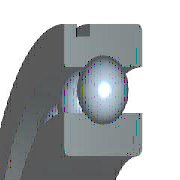
# Autodesk Inventor part: 滚动轴承 6200 N GB/T 276-94
Saved by Autodesk Inventor 2015 (Build 190159000, 159)
## iProperties
Created: 2014-02-16
Part Number: 滚动轴承 6200 N GB/T 276-94
Material: 钢，软
Description: 滚动轴承 - 深沟球轴承 - 外形尺寸
Document SubType Name: Modeling
Standard: GB/T 276-1994
Designer: Administrator
Standard Revision: 1994
Standards Organization: GB
Language: zh-CN
Size Designation: 6200 N
Categories: <MemberInstance><Categories><Category DisplayName="轴用零件" InternalName="7f7aeb1f-a693-4053-b835-cee3144e0d98" Mnemonic="SHFT"><Category DisplayName="轴承" InternalName="242d30a3-7172-44e6-a363-b0a3d8f1b556" Mnemonic="BRNG"><CategoryParameter DisplayName="宽度" InternalName="25fc5f6e-338b-4801-b5ed-8959743e396e" Mnemonic="wdth"/><CategoryParameter DisplayName="尺寸规格" InternalName="2c4e891a-c8f4-49ed-a5c1-5131476c6feb" Mnemonic="sizedes"/><CategoryParameter DisplayName="额定基本动态载荷" InternalName="440972dd-7009-4861-bd45-69ffbb461423" Mnemonic="bdynlrat"/><CategoryParameter DisplayName="轴直径" InternalName="91302473-2833-4451-a660-c5d4a8d6a031" Mnemonic="shaftdia"/><CategoryParameter DisplayName="接触角" InternalName="aa21a452-7974-4a55-b5cf-1c2972de2aea" Mnemonic="TouchAngle"/><CategoryParameter DisplayName="外径" InternalName="d441686c-04bd-4681-b674-94fbc173ec23" Mnemonic="outdia"/><Category DisplayName="球轴承" InternalName="9b553946-0899-4a5e-a403-c1d9295e77c1" Mnemonic="BALLBEAR"><CategoryParameter DisplayName="当 Fa/Fr &lt;= e 时的径向动态载荷系数" InternalName="051e59b3-bd55-4dad-8b07-38b5cb912881" Mnemonic="raddynfc1"/><CategoryParameter DisplayName="基本额定静载荷" InternalName="0f13fbbf-c511-4d43-b4c7-197b47424baf" Mnemonic="bstatlrat"/><CategoryParameter DisplayName="确定寿命的指数" InternalName="3029e2ef-9460-4be8-bdfd-dfe61437473d" Mnemonic="lifeexp"/><CategoryParameter DisplayName="摩擦系数" InternalName="3086b0f2-3d69-46ff-8a75-fe12e395bb47" Mnemonic="fricfct"/><CategoryParameter DisplayName="最小轴径" InternalName="4a5be9bc-ad86-4bf2-8167-102dad5d3e27" Mnemonic="minshaftdia"/><CategoryParameter DisplayName="当 Fa/Fr &gt; e 时的轴向动态载荷系数" InternalName="4b6ff741-5956-4a40-80f5-34eb9259f88c" Mnemonic="axdynfc2"/><CategoryParameter DisplayName="极限速度 (润滑脂)" InternalName="5237843b-2c8d-46d3-8227-f3e9dd85a12e" Mnemonic="lubgrsp"/><CategoryParameter DisplayName="极限速度 (润滑油)" InternalName="60628548-8907-44dc-8e09-603d72f5766f" Mnemonic="oilspd"/><CategoryParameter DisplayName="轴向静态载荷系数" InternalName="74dbf5e2-8362-409a-802f-3c2235668d99" Mnemonic="axdynfc0"/><CategoryParameter DisplayName="质量" InternalName="7b80f85c-da81-4dea-b8db-d7c689da91b2" Mnemonic="mass"/><CategoryParameter DisplayName="半径" InternalName="83352640-dfae-4cba-bc9f-11ecbfb0001c" Mnemonic="rad"/><CategoryParameter DisplayName="径向静态载荷系数" InternalName="83ce084d-c51e-4598-a871-e8e1e34b26ee" Mnemonic="raddynfc0"/><CategoryParameter DisplayName="当 Fa/Fr &lt;= e 时的轴向动态载荷系数" InternalName="ae45a7db-08df-4411-99a8-2f035015bff9" Mnemonic="axdynfc1"/><CategoryParameter DisplayName="最大安装孔肩直径" InternalName="b5cf89e0-ca87-439c-b08c-a25e2999ab06" Mnemonic="maxhubdia"/><CategoryParameter DisplayName="确定系数的极限值" InternalName="be0ce6fc-cad4-4218-b484-c34dd2571812" Mnemonic="limvalfac"/><CategoryParameter DisplayName="当 Fa/Fr &gt; e 时的径向动态载荷系数" InternalName="e513bdb7-139f-4b3c-af32-49e0ba1226b9" Mnemonic="raddynfc2"/><CategoryParameter DisplayName="最大阶梯圆角半径" InternalName="f6ce6695-cf2c-4ec9-8d20-66671e0e35a4" Mnemonic="maxstprad"/><Category DisplayName="深沟球轴承" InternalName="6f040212-0f73-4fa8-b5e4-17d6525fdc38" Mnemonic="BBDGBB"/></Category></Category></Category><Category DisplayName="数据类型" InternalName="23b78d0f-2648-40c6-8793-ca6db495c9e8" Mnemonic="DATATYPE"><CategoryParameter DisplayName="显示名" InternalName="05415f3d-3907-474b-a020-eb9d644f4cf3" Mnemonic="DISPLAYNAME"/><CategoryParameter DisplayName="标准" InternalName="0c0a119c-1e12-4c84-803f-101930972f5e" Mnemonic="STANDARD"/><CategoryParameter DisplayName="描述" InternalName="13903e3d-64b1-4950-80da-f627842ea37f" Mnemonic="DESCRIPTION"/><CategoryParameter DisplayName="规格" InternalName="2675968c-4ce5-49e0-a4f5-552d29089031" Mnemonic="DESIGNATION"/><CategoryParameter DisplayName="默认列" InternalName="2af9ec52-faaa-4026-b378-f9fa4afca842" Mnemonic="DEFAULTROW"/><CategoryParameter DisplayName="文件夹名称" InternalName="3f06958e-8713-4116-9be7-ed6184ecc97b" Mnemonic="FOLDERNAME"/><CategoryParameter DisplayName="版本指南" InternalName="45a75005-10b1-4dfc-8d6d-dfe629f0b93c" Mnemonic="REVISIONGUID"/><CategoryParameter DisplayName="文件名" InternalName="8b46a4cc-9585-4fed-90c3-899f57e09a73" Mnemonic="FILENAME"/><CategoryParameter DisplayName="标准组织" InternalName="8f5914e1-4693-403f-8ab5-d37768198c9d" Mnemonic="STDSORG"/><CategoryParameter DisplayName="系列版本" InternalName="914462f6-6e19-4b14-ba84-155b9680b1d0" Mnemonic="FAMILYREVISION"/><CategoryParameter DisplayName="标准版本" InternalName="91d5a463-65c2-4fde-b823-3b7fea5e8e17" Mnemonic="STANDARDREVISION"/><CategoryParameter DisplayName="成员版本" InternalName="a65d44b9-392f-4f4f-857b-e4b3d54996fe" Mnemonic="MEMBERREVISION"/><CategoryParameter DisplayName="剪裁格式" InternalName="bc51e27b-3422-4e78-93ef-cec197ddf230" Mnemonic="CLIPFORMAT"/><CategoryParameter DisplayName="制造商" InternalName="cd6c7a72-a28a-4e50-99a9-2c7f4e13e5ad" Mnemonic="MANUFACTURER"/><CategoryParameter DisplayName="内部名称" InternalName="cf1d0246-76d9-4b4a-8305-fa0409afb5c1" Mnemonic="INTERNALNAME"/><CategoryParameter DisplayName="是否公制" InternalName="e2385c5b-1ea4-4823-96a8-8de651266ec3" Mnemonic="ISMETRIC"/><Category DisplayName="零件" InternalName="c0e0b642-3bcb-4cc8-9e80-f96d35c4afa4" Mnemonic="PART"><CategoryParameter DisplayName="零件代号" InternalName="016b6077-bfbe-49bd-92c9-d8d59c39c941" Mnemonic="PARTNUMBER"/><CategoryParameter DisplayName="库存编号" InternalName="4dba7c1c-e26c-444e-836c-b08b433409a8" Mnemonic="STOCKNUMBER"/><CategoryParameter DisplayName="材料键" InternalName="5c9a8adb-dd2b-4535-b97f-0a94a95fe41f" Mnemonic="MATERIALKEY"/><CategoryParameter DisplayName="材料" InternalName="818a152a-d3c3-49ca-80ee-df7d91421b8e" Mnemonic="MATERIAL"/></Category></Category><Category DisplayName="先前版本映射" InternalName="cd87c42b-3e48-431e-b5c0-1cbeb14dfe77" Mnemonic="LEGACYMAP"><CategoryParameter DisplayName="唯一 DA 成员 ID" InternalName="0918ad47-427f-4fed-ae26-24c81c58f590" Mnemonic="DACOOKIE"/><CategoryParameter DisplayName="合并11 ID" InternalName="0ee8fb18-e2ed-4f39-96f6-1f4b5f50aa71" Mnemonic="MERGE11"/><CategoryParameter DisplayName="唯一 CC 成员 ID" InternalName="5193edd4-b2b0-4ab4-9d54-de900eee34e0" Mnemonic="CCCOOKIE"/><CategoryParameter DisplayName="分割 ID" InternalName="72b5c83c-be7f-45c4-ae51-9160ea6deb26" Mnemonic="SPLIT"/><CategoryParameter DisplayName="成员 ID" InternalName="8e5e0294-fc51-4c8f-b3d7-003dc5ed94f6" Mnemonic="MEMBERID"/><CategoryParameter DisplayName="目录名" InternalName="d99d1e27-aa94-4de2-af4c-c348882a6f4f" Mnemonic="CATALOGNAME"/><CategoryParameter DisplayName="系列编号" InternalName="e705e1f4-09cb-413e-91f9-551b4188271e" Mnemonic="FAMILYNUMBER"/></Category></Categories><FamilyTemplate Id="br1000"><FamilyTemplateParameters><FamilyTemplateParameter ObjectType="kUserParameterObject" ValueType="xs:double" Id="1" ObjectReferenceKey="WR"/><FamilyTemplateParameter ObjectType="kUserParameterObject" ValueType="xs:double" Id="2" ObjectReferenceKey="BC"/><FamilyTemplateParameter ObjectType="kUserParameterObject" ValueType="xs:double" Id="3" ObjectReferenceKey="ND"/><FamilyTemplateParameter ObjectType="kUserParameterObject" ValueType="xs:double" Id="4" ObjectReferenceKey="KR1S"/><FamilyTemplateParameter ObjectType="kUserParameterObject" ValueType="xs:double" Id="5" ObjectReferenceKey="KRS"/><FamilyTemplateParameter ObjectType="kUserParameterObject" ValueType="xs:double" Id="6" ObjectReferenceKey="WD"/><FamilyTemplateParameter ObjectType="kUserParameterObject" ValueType="xs:double" Id="7" ObjectReferenceKey="ND2"/><FamilyTemplateParameter ObjectType="kUserParameterObject" ValueType="xs:double" Id="8" ObjectReferenceKey="NBR"/><FamilyTemplateParameter ObjectType="kUserParameterObject" ValueType="xs:double" Id="9" ObjectReferenceKey="KB"/><FamilyTemplateParameter ObjectType="kUserParameterObject" ValueType="xs:double" Id="10" ObjectReferenceKey="RT"/><FamilyTemplateParameter ObjectType="kUserParameterObject" ValueType="xs:double" Id="11" ObjectReferenceKey="BC0"/><FamilyTemplateParameter ObjectType="kUserParameterObject" ValueType="xs:double" Id="12" ObjectReferenceKey="BD"/><FamilyTemplateParameter ObjectType="kUserParameterObject" ValueType="xs:double" Id="13" ObjectReferenceKey="NBR2"/><FamilyTemplateParameter ObjectType="kUserParameterObject" ValueType="xs:double" Id="14" ObjectReferenceKey="NBR3"/><FamilyTemplateParameter ObjectType="kUserParameterObject" ValueType="xs:double" Id="15" ObjectReferenceKey="BR"/><FamilyTemplateParameter ObjectType="kUserParameterObject" ValueType="xs:double" Id="16" ObjectReferenceKey="BI"/><FamilyTemplateParameter ObjectType="kPropertyObject" ValueType="xs:string" Id="100" ObjectReferenceKey="{32853F0F-3444-11d1-9E93-0060B03C1CA6}" SubObjectId="52"/><FamilyTemplateParameter ObjectType="kPropertyObject" ValueType="xs:string" Id="105" ObjectReferenceKey="{32853F0F-3444-11d1-9E93-0060B03C1CA6}" SubObjectId="5"/><FamilyTemplateParameter ObjectType="kPartComponentDefinitionObject" ValueType="xs:string" Id="110" SubObjectId="Material"/></FamilyTemplateParameters></FamilyTemplate><CategoryParameterMap><ParamToTemplateMap><ParamToTemplate CategoryParameter="//CategoryParameter[@InternalName='05415f3d-3907-474b-a020-eb9d644f4cf3']" ConstantValue="Rolling bearing GB/T 276-1994 Type 60000 N"/><ParamToTemplate CategoryParameter="//CategoryParameter[@InternalName='cf1d0246-76d9-4b4a-8305-fa0409afb5c1']" ConstantValue="7bafe8d5-59fe-490f-b763-b71ca55f5a5a"/><ParamToTemplate CategoryParameter="//CategoryParameter[@InternalName='3f06958e-8713-4116-9be7-ed6184ecc97b']" ConstantValue="GB_T 276-94  (60000 N)"/><ParamToTemplate CategoryParameter="//CategoryParameter[@InternalName='914462f6-6e19-4b14-ba84-155b9680b1d0']" ConstantValue="10"/><ParamToTemplate CategoryParameter="//CategoryParameter[@InternalName='bc51e27b-3422-4e78-93ef-cec197ddf230']" ConstantValue="CF_INVENTOR.STDPARTS"/><ParamToTemplate CategoryParameter="//CategoryParameter[@InternalName='e2385c5b-1ea4-4823-96a8-8de651266ec3']" ConstantValue="true"/><ParamToTemplate CategoryParameter="//CategoryParameter[@InternalName='13903e3d-64b1-4950-80da-f627842ea37f']" ConstantValue="Rolling bearings - Deep groove ball bearings - Boundary dimensions"/><ParamToTemplate CategoryParameter="//CategoryParameter[@InternalName='8f5914e1-4693-403f-8ab5-d37768198c9d']" ConstantValue="GB"/><ParamToTemplate CategoryParameter="//CategoryParameter[@InternalName='0c0a119c-1e12-4c84-803f-101930972f5e']" ConstantValue="GB/T 276-1994"/><ParamToTemplate CategoryParameter="//CategoryParameter[@InternalName='cd6c7a72-a28a-4e50-99a9-2c7f4e13e5ad']" TemplateParameter="104"/><ParamToTemplate CategoryParameter="//CategoryParameter[@InternalName='91d5a463-65c2-4fde-b823-3b7fea5e8e17']" ConstantValue="1994"/><ParamToTemplate CategoryParameter="//CategoryParameter[@InternalName='45a75005-10b1-4dfc-8d6d-dfe629f0b93c']" ConstantValue="e7965a8e-b613-47da-b247-244c6e5a2f40"/><ParamToTemplate CategoryParameter="//CategoryParameter[@InternalName='2af9ec52-faaa-4026-b378-f9fa4afca842']" ConstantValue="10"/><ParamToTemplate CategoryParameter="//CategoryParameter[@InternalName='d99d1e27-aa94-4de2-af4c-c348882a6f4f']" ConstantValue="GB"/><ParamToTemplate CategoryParameter="//CategoryParameter[@InternalName='e705e1f4-09cb-413e-91f9-551b4188271e']" ConstantValue="234"/><ParamToTemplate CategoryParameter="//CategoryParameter[@InternalName='8b46a4cc-9585-4fed-90c3-899f57e09a73']" ConstantValue="滚动轴承 6200 N GB/T 276-94"/><ParamToTemplate CategoryParameter="//CategoryParameter[@InternalName='a65d44b9-392f-4f4f-857b-e4b3d54996fe']" ConstantValue="70b880fe-f15a-4bed-88e7-ae4e282b28b7"/><ParamToTemplate CategoryParameter="//CategoryParameter[@InternalName='2c4e891a-c8f4-49ed-a5c1-5131476c6feb']" ConstantValue="6200 N"/><ParamToTemplate CategoryParameter="//CategoryParameter[@InternalName='8e5e0294-fc51-4c8f-b3d7-003dc5ed94f6']" ConstantValue="200"/><ParamToTemplate CategoryParameter="//CategoryParameter[@InternalName='d441686c-04bd-4681-b674-94fbc173ec23']" TemplateParameter="12"/><ParamToTemplate CategoryParameter="//CategoryParameter[@InternalName='2675968c-4ce5-49e0-a4f5-552d29089031']" TemplateParameter="100"/><ParamToTemplate CategoryParameter="//CategoryParameter[@InternalName='25fc5f6e-338b-4801-b5ed-8959743e396e']" TemplateParameter="9"/><ParamToTemplate CategoryParameter="//CategoryParameter[@InternalName='83352640-dfae-4cba-bc9f-11ecbfb0001c']" TemplateParameter="5"/><ParamToTemplate CategoryParameter="//CategoryParameter[@InternalName='818a152a-d3c3-49ca-80ee-df7d91421b8e']" TemplateParameter="110"/><ParamToTemplate CategoryParameter="//CategoryParameter[@InternalName='016b6077-bfbe-49bd-92c9-d8d59c39c941']" TemplateParameter="105"/><ParamToTemplate CategoryParameter="//CategoryParameter[@InternalName='91302473-2833-4451-a660-c5d4a8d6a031']" TemplateParameter="6"/></ParamToTemplateMap></CategoryParameterMap></MemberInstance>
Density: 1 g/cm^3
Appearance: 半抛光
IsCustomPart: 0
Author: Administrator
Autodesk Inventor part; units mm, degrees
note: some values were not read from the file. Left out: dimensions or parameters whose unit could not be read.
ref_plane "YZ Plane" through (0, 0, 0) normal (1, 0, 0) x (0, 1, 0)
ref_plane "XZ Plane" through (0, 0, 0) normal (0, 1, 0) x (-1, 0, 0)
ref_plane "XY Plane" through (0, 0, 0) normal (0, 0, 1) x (1, 0, 0)
sketch "草图" plane through (0, 0, 0) normal (0, 0, 1) x (1, 0, 0)
  circle A0 centre (4.5, 10) radius 2.6
  line L0 (4.5, 10) -> (7.1, 10)
  line L1 (4.5, 10) -> (1.9, 10)
  line L2 (4.5, 7.4) -> (4.5, 12.6)
  line L3 (2.568058, 8.26) -> (0, 8.26)
  line L4 (0, 8.26) -> (0, 8.26)
  line L5 (0, 8.26) -> (0, 8.26)
  line L6 (0, 5) -> (9, 5)
  line L7 (2.568058, 11.74) -> (0, 11.74)
  line L8 (0, 11.74) -> (0, 11.74)
  line L9 (0, 11.74) -> (0, 11.74)
  line L10 (0, 15) -> (1.5, 15)
  line L11 (1.5, 15) -> (1.5, 13.92)
  line L12 (1.5, 13.92) -> (3, 13.92)
  line L13 (3, 13.92) -> (3, 15)
  line L14 (3, 15) -> (9, 15)
  line L15 (6.431942, 8.26) -> (9, 8.26)
  line L16 (9, 8.26) -> (9, 8.26)
  line L17 (9, 8.26) -> (9, 8.26)
  line L18 (9, 8.26) -> (9, 5)
  line L19 (6.431942, 11.74) -> (9, 11.74)
  line L20 (9, 11.74) -> (9, 11.74)
  line L21 (9, 11.74) -> (9, 11.74)
  line L22 (9, 11.74) -> (9, 15)
  line L23 (-3, 0) -> (18, 0)
  line L24 (0, -1.2) -> (0, 10.7)
  line L25 (0, 11.74) -> (0, 11.74)
  line L26 (0, 11.74) -> (0, 11.74)
  line L27 (0, 8.26) -> (0, 8.26)
  line L28 (0, 8.26) -> (0, 8.26)
  line L29 (9, 11.74) -> (9, 11.74)
  line L30 (9, 11.74) -> (9, 11.74)
  line L31 (9, 8.26) -> (9, 8.26)
  line L32 (9, 8.26) -> (9, 8.26)
  dimension "d0" = 5.2
  dimension "d7" = 10
  dimension "d8" = 30
  dimension "d9" = 20
  dimension "d10" = 27.84
  dimension "d11" = 16.52
  dimension "d12" = 16.52
  dimension "d13" = 16.52
  dimension "d14" = 0
  dimension "d15" = 9
  dimension "d16" = 9
  dimension "d19" = 1.5
  dimension "d20" = 3
  dimension "d22" = 4.5
  constraints: 62 end point, 9 perpendicular, 9 point on line, 7 symmetric about line, 5 parallel, 4 collinear, 1 midpoint, 20 other
  measures "d7" diameter of L6 L23
  measures "d8" diameter of L10 L23
  measures "d9" diameter of L0.start L23
  measures "d10" diameter of L12 L23
  measures "d11" diameter of L28 L23
  measures "d12" diameter of L32 L23
  measures "d13" diameter of L3 L23
  measures "d14" distance between parallel lines of L24 L27
  measures "d15" distance between parallel lines of L24 L29
  measures "d16" distance between parallel lines of L24 L18
  measures "d19" distance between parallel lines of L24 L11
  measures "d20" distance between parallel lines of L24 L13
  measures "d22" distance from line of L24 L0.start
sketch "草图 outline for 轴承体" plane through (0, 0, 0) normal (0, 0, 1) x (1, 0, 0)
  arc A0 (2.568058, 11.74) -> (6.431942, 11.74) centre (4.5, 10) cw
  line L0 (6.431942, 11.74) -> (9, 11.74)
  line L1 (9, 11.74) -> (9, 15)
  line L2 (9, 15) -> (3, 15)
  line L3 (3, 15) -> (3, 13.92)
  line L4 (3, 13.92) -> (1.5, 13.92)
  line L5 (1.5, 13.92) -> (1.5, 15)
  line L6 (1.5, 15) -> (0, 15)
  line L7 (0, 15) -> (0, 11.74)
  line L8 (0, 11.74) -> (2.568058, 11.74)
  arc A1 (6.431942, 8.26) -> (2.568058, 8.26) centre (4.5, 10) cw
  line L9 (2.568058, 8.26) -> (0, 8.26)
  line L10 (0, 8.26) -> (0, 5)
  line L11 (0, 5) -> (9, 5)
  line L12 (9, 5) -> (9, 8.26)
  line L13 (9, 8.26) -> (6.431942, 8.26)
revolve "轴承体" add sketch "草图 outline for 轴承体" angle 360 about axis through (-10, 0, 0) along (1, 0, 0)
fillet "圆角1" radius 0.6 4 edges at (0, -15, 0) (9, -15, 0) (0, -5, 0) (9, -5, 0)
revolve "球" add sketch "草图" angle 360 about axis through (4.5, 10, 0) along (-1, 0, 0) picked at (6.106098, 10.616648) picked at (2.79242, 10.209703) contours L0 L2 A0 | L1 A0 L2
pattern_circular "IDS_ARRAYBALL[SIMPL:T]" count 6 over 360 about axis through (-10, 0, 0) along (1, 0, 0) of "球"
equation "\"d0\" = -0.26 * WD + 0.26 * BD"
equation "\"d7\" = WD"
equation "\"d8\" = BD"
equation "\"d9\" = 0.5 * WD + 0.5 * BD"
equation "\"d10\" = BD - 2 * RT"
equation "\"d11\" = ND2"
equation "\"d12\" = ND"
equation "\"d13\" = 0.326 * BD + 0.674 * WD"
equation "\"d15\" = KB - NBR"
equation "\"d16\" = KB"
equation "\"d19\" = NBR3"
equation "\"d20\" = 2 * NBR3"
equation "\"d22\" = 0.5 * KB"
equation "\"d1\" = KRS"
equation "\"WD\" = 10"
equation "\"BD\" = 30"
equation "\"KB\" = 9"
equation "\"KRS\" = 0.6"
equation "\"ND\" = 0.674 * WD + 0.326 * BD"
equation "\"ND2\" = 0.674 * WD + 0.326 * BD"
equation "\"NBR2\" = 0"
equation "\"RT\" = 1.8 * KRS"
equation "\"NBR\" = 0"
equation "\"NBR3\" = 0.166667 * KB"
equation "\"WR\" = 0.5 * WD"
equation "\"KR1S\" = 0.5"
equation "\"BR\" = 0.5 * BD"
body "Solid1"
